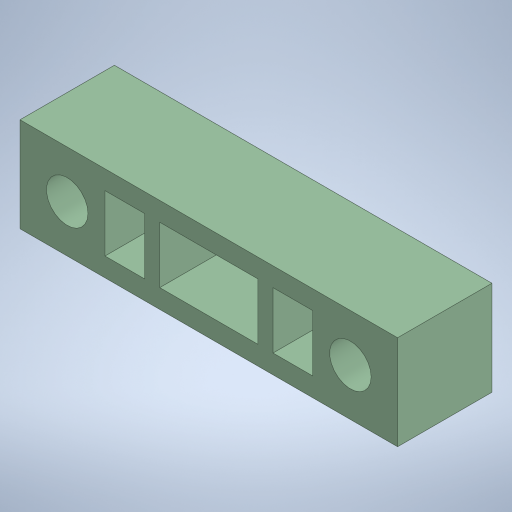
# Autodesk Inventor part: griper_TPU
Saved by Autodesk Inventor 2024 (Build 280153000, 153)
## iProperties
Created: 2025-06-02
Part Number: griper_TPU
Material: ゴム、シリコーン
Document SubType Name: Modeling
Designer: 1412z
Density: 1.25 g/cm^3
Appearance: ゴム - 緑
Author: 1412z
Autodesk Inventor part; units mm, degrees
ref_plane "YZ Plane" through (0, 0, 0) normal (1, 0, 0) x (0, 1, 0)
ref_plane "XZ Plane" through (0, 0, 0) normal (0, 1, 0) x (-1, 0, 0)
ref_plane "XY Plane" through (0, 0, 0) normal (0, 0, 1) x (1, 0, 0)
sketch "スケッチ1" plane through (0, 0, 0) normal (0, 0, 1) x (1, 0, 0)
  line L0 (10, -2.5) -> (-10, -2.5)
  line L1 (-10, -2.5) -> (-10, 2.5)
  line L2 (-10, 2.5) -> (10, 2.5)
  line L3 (10, 2.5) -> (10, -2.5)
  line L4 (10, -2.5) -> (-10, 2.5) construction
  line L5 (-10, -2.5) -> (10, 2.5) construction
  circle A0 centre (-7.5, 0) radius 1.1
  circle A1 centre (7.5, 0) radius 1.1
  line L6 (5.5, -2.5) -> (5.5, 2.5)
  line L7 (-5.5, 2.5) -> (-5.5, -2.5)
  line L8 (-5.5, -1.5) -> (5.5, -1.5)
  line L9 (-5.5, 1.5) -> (5.5, 1.5)
  line L10 (3, -1.5) -> (3, 1.5)
  line L11 (3, 1.5) -> (3.4, 1.5)
  line L12 (3.4, 1.5) -> (3.4, -1.5)
  line L13 (3, -1.5) -> (2.6, -1.5)
  line L14 (2.6, -1.5) -> (2.6, 1.5)
  line L15 (-3, -1.5) -> (-3, 1.5)
  line L16 (-3, 1.5) -> (-3.4, 1.5)
  line L17 (-3.4, 1.5) -> (-3.4, -1.5)
  line L18 (-3, -1.5) -> (-2.6, -1.5)
  line L19 (-2.6, -1.5) -> (-2.6, 1.5)
  point P0 (0, 0)
  dimension "d0" = 20
  dimension "d1" = 5
  dimension "d2" = 2.2
  dimension "d3" = 2.2
  dimension "d4" = 0.4
  dimension "d5" = 0.4
  dimension "d6" = 0.4
  dimension "d7" = 0.4
  dimension "d10" = 1
  dimension "d11" = 1
  constraints: 40 end point, 20 point on line, 11 perpendicular, 2 centre point, 2 midpoint, 2 parallel, 1 horizontal
  measures "d0" distance of L1.end L2.end
  measures "d1" distance of L0.end L1.end
  measures "d2" diameter of A0
  measures "d3" diameter of A1
  measures "d4" distance of L10.end L11.end
  measures "d5" distance of L10.start L13.end
  measures "d6" distance of L15.end L16.end
  measures "d7" distance of L15.start L18.end
  measures "d10" distance between parallel lines of L9 L2
  measures "d11" distance between parallel lines of L0 L8
extrude "押し出し1" add sketch "スケッチ1" along normal blind 5 contours L0 L6 L2 L3 | L0 L7 L8 L6 | L0 L1 L2 L7 | L6 L9 L7 L2 | L8 L10 L9 L12 | L17 L9 L15 L8 | L8 L14 L9 L10 | L15 L9 L19 L8
